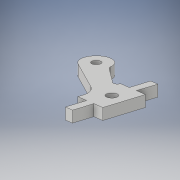
# Autodesk Inventor part: 小零件3
Saved by Autodesk Inventor 2017 (Build 210142000, 142)
## iProperties
Part Number: 小零件3
Material: 一般
Document SubType Name: Modeling
Designer: User
Density: 1 g/cm^3
Appearance: 預設
Author: User
Autodesk Inventor part; units mm, degrees
ref_plane "YZ Plane" through (0, 0, 0) normal (1, 0, 0) x (0, 1, 0)
ref_plane "XZ Plane" through (0, 0, 0) normal (0, 1, 0) x (-1, 0, 0)
ref_plane "XY Plane" through (0, 0, 0) normal (0, 0, 1) x (1, 0, 0)
sketch "草圖1" plane through (0, 0, 0) normal (0, 1, 0) x (-1, 0, 0)
  line L0 (4.2304, -5.8965) -> (4.2304, -5.9439)
  line L1 (4.2304, -5.9439) -> (0.0304, -5.9439)
  line L2 (0.0304, -5.9439) -> (1.2304, -5.9439)
  line L3 (1.2304, -5.9439) -> (1.2304, -11.9439)
  line L4 (1.2304, -11.9439) -> (0.0304, -11.9439)
  line L5 (-4.1696, 0.0561) -> (-4.1696, -5.9439)
  line L6 (-4.1696, -5.9439) -> (0.0304, -5.9439)
  line L7 (0.0304, -5.9439) -> (-1.1696, -5.9439)
  line L8 (-1.1696, -5.9439) -> (-1.1696, -11.9439)
  line L9 (-1.1696, -11.9439) -> (0.0304, -11.9439)
  line L10 (4.2304, 4.5332) -> (4.2304, 6.0561)
  line L11 (4.2304, 6.0561) -> (0.0304, 6.0561)
  line L12 (0.0304, 6.0561) -> (1.2304, 6.0561)
  line L13 (1.2304, 6.0561) -> (1.2304, 12.0561)
  line L14 (1.2304, 12.0561) -> (0.0304, 12.0561)
  line L15 (-4.1696, 0.0561) -> (-4.1696, 6.0561)
  line L16 (-4.1696, 6.0561) -> (0.0304, 6.0561)
  line L17 (0.0304, 6.0561) -> (-1.1696, 6.0561)
  line L18 (-1.1696, 6.0561) -> (-1.1696, 12.0561)
  line L19 (-1.1696, 12.0561) -> (0.0304, 12.0561)
  circle A0 centre (0, 0) radius 1.5
  circle A1 centre (17.1565, -10) radius 1.25
  arc A2 (13.2007, -10.5927) -> (19.0627, -6.4834) centre (17.1565, -10) ccw
  line L20 (19.0627, -6.4834) -> (6.8478, 0.1374)
  line L21 (12.7818, -9.9193) -> (5.8005, -5.075)
  arc A3 (4.2304, 4.5332) -> (6.8478, 0.1374) centre (9.2304, 4.5332) ccw
  arc A4 (5.8005, -5.075) -> (4.2304, -5.8965) centre (5.2304, -5.8965) ccw
  arc A5 (13.2007, -10.5927) -> (12.7818, -9.9193) centre (12.2117, -10.7409) ccw
  point P0 (4.2304, 0.0561)
  point P1 (13.1607, -10.1822)
  dimension "d0" = 6
  dimension "d1" = 1.2
  dimension "d2" = 3
  dimension "d3" = 6
  dimension "d4" = 3
  dimension "d9" = 2.5
  dimension "d10" = 8
  dimension "d11" = 5
  dimension "d12" = 1
  dimension "d13" = 1
  constraints: 44 end point, 9 point on circle, 7 tangent, 6 centre point, 3 point on line, 2 coincident, 1 horizontal, 1 parallel, 1 perpendicular, 1 other
  measures "d0" distance of point (4.23, 0.056) L0.end
  measures "d1" distance of L3.end L4.end
  measures "d2" distance between parallel lines of L3 L0
  measures "d3" distance of L2.end L3.end
  measures "d4" diameter of A0
  measures "d9" diameter of A1
  measures "d10" diameter of A2
  measures "d11" radius of A3
  measures "d12" radius of A4
  measures "d13" radius of A5
extrude "擠出1" add sketch "草圖1" along normal mid plane 3
